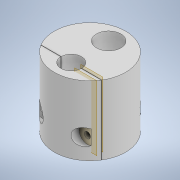
# Autodesk Inventor part: small_actuator_holder
Saved by Autodesk Inventor 2021 (Build 250183000, 183)
## iProperties
Created: 2020-10-24
Part Number: small_actuator_holder
Material: Generic
Document SubType Name: Modeling
Designer: bober
Density: 1 g/cm^3
Appearance: Default
Author: bober
Autodesk Inventor part; units mm, degrees
ref_plane "YZ Plane" through (0, 0, 0) normal (1, 0, 0) x (0, 1, 0)
ref_plane "XZ Plane" through (0, 0, 0) normal (0, 1, 0) x (-1, 0, 0)
ref_plane "XY Plane" through (0, 0, 0) normal (0, 0, 1) x (1, 0, 0)
sketch "Sketch1" plane through (0, 0, 0) normal (0, 1, 0) x (-1, 0, 0)
  circle A0 centre (0, 0) radius 17.5
  line L0 (-9.1924, 0) -> (0, 9.1924)
  line L1 (0, 9.1924) -> (9.1924, 0)
  line L2 (9.1924, 0) -> (0, -9.1924)
  line L3 (0, -9.1924) -> (-9.1924, 0)
  line L4 (-6.5, 6.5) -> (6.5, -6.5) construction
  line L5 (6.5, 6.5) -> (-6.5, -6.5) construction
  circle A1 centre (0, 9.1924) radius 5.045
  circle A2 centre (0, -9.1924) radius 6
  line L6 (-18.2848, 9.2924) -> (18.2848, 9.2924)
  line L7 (18.2848, 9.2924) -> (18.2848, 9.0924)
  line L8 (18.2848, 9.0924) -> (-18.2848, 9.0924)
  line L9 (-18.2848, 9.0924) -> (-18.2848, 9.2924)
  line L10 (-18.2848, 9.2924) -> (18.2848, 9.0924) construction
  line L11 (18.2848, 9.2924) -> (-18.2848, 9.0924) construction
  point P0 (5.044, 9.2924)
  point P1 (14.8291, 9.2924)
  point P2 (-14.8291, 9.2924)
  point P3 (-5.044, 9.2924)
  point P4 (-5.044, 9.0924)
  point P5 (-14.9525, 9.0924)
  point P6 (14.9525, 9.0924)
  point P7 (5.044, 9.0924)
  dimension "d0" = 35
  dimension "d1" = 13
  dimension "d2" = 13
  dimension "d3" = 10.09
  dimension "d4" = 12
  dimension "d5" = 0.2
  constraints: 24 end point, 4 midpoint, 4 parallel, 3 centre point, 3 coincident, 2 perpendicular, 1 horizontal
  measures "d0" diameter of A0
  measures "d1" distance of L1.end L2.end
  measures "d2" distance of L0.end L1.end
  measures "d3" diameter of A1
  measures "d4" diameter of A2
  measures "d5" distance of L6.end L7.end
extrude "Extrusion1" add sketch "Sketch1" along normal blind 29 contours A0 L8 A1 L0 L3 A2 L2 L1 | L6 A1 A0 | L1 L2 A2 L3 L0 A1
sketch "Sketch2" plane through (14.8291, 0, 9.2924) normal (0, 0, -1) x (-1, 0, 0)
  circle A0 centre (4, 5) radius 1.5
  point P0 (14.8291, 0)
  dimension "d8" = 3
  constraints: 1 centre point
  measures "d8" diameter of A0
hole "Hole1" at (10.8291, 5, 9.2924) direction (0, 0, 1) diameter 3 end through all both
sketch "Sketch3" plane through (14.8291, 0, 9.2924) normal (0, 0, -1) x (-1, 0, 0)
  circle A0 centre (4, 5) radius 1.5 projected
  point P0 (14.8291, 0)
  constraints: 1 coincident
ref_plane "Work Plane1" through (5.044, 0, -5.9076) normal (0, 0, 1) x (1, 0, 0)
sketch "Sketch4" plane through (5.044, 0, -5.9076) normal (0, 0, 1) x (1, 0, 0)
  circle A0 centre (5.7851, 5) radius 1.5 projected
  circle A1 centre (5.7851, 5) radius 2.75
  line L0 (3.0351, 6.5877) -> (5.7851, 8.1754)
  line L1 (5.7851, 8.1754) -> (8.5351, 6.5877)
  line L2 (8.5351, 6.5877) -> (8.5351, 3.4123)
  line L3 (8.5351, 3.4123) -> (5.7851, 1.8246)
  line L4 (5.7851, 1.8246) -> (3.0351, 3.4123)
  line L5 (3.0351, 3.4123) -> (3.0351, 6.5877)
  point P0 (-5.044, 0)
  point P1 (3.0351, 5)
  dimension "d17" = 5.5
  constraints: 12 end point, 2 coincident, 1 horizontal alignment, 1 midpoint, 15 other
extrude "Extrusion2" cut sketch "Sketch4" against normal blind 19 contours A0 | A1 | L2 L3 A1 | A1 L1 L2 | A1 L0 L1 | L3 L4 A1 | A1 L5 L0 | L4 L5 A1
mirror "Mirror1" about plane through (0, 0, 0) normal (1, 0, 0) of "Hole1", "Extrusion2"
ref_plane "Work Plane2" through (5.044, 0, 9.0924) normal (0, 0, 1) x (1, 0, 0)
ref_plane "Work Plane3" through (5.044, 0, 12.0924) normal (0, 0, 1) x (1, 0, 0)
sketch "Sketch5" plane through (5.044, 0, 12.0924) normal (0, 0, 1) x (1, 0, 0)
  circle A0 centre (5.7851, 5) radius 1.5 projected
  circle A1 centre (5.7851, 5) radius 4
  circle A2 centre (-15.8731, 5) radius 1.5 projected
  circle A3 centre (-15.8731, 5) radius 4
  point P0 (-5.044, 0)
  dimension "d26" = 8
  dimension "d27" = 8
  constraints: 2 centre point, 2 coincident
  measures "d26" diameter of A1
  measures "d27" diameter of A3
thicken "Thicken3" operation add thickness 5 both sides no extend neighbours yes toward (0, -1, 0) faces at (10.7531, 0, 10.3158)
thicken "Thicken4" operation add thickness 5 both sides no extend neighbours yes toward (0, -1, 0) faces at (-8.5704, 0, 0.4787)
extrude "Extrusion3" cut sketch "Sketch5" along normal blind 10
split body "Split2" result two bodies by plane through (5.044, 0, 9.0924) normal (0, 0, 1) first body at (3.5258, 9.7972, 16.6304)
body "Solid4"
body "Solid5"
